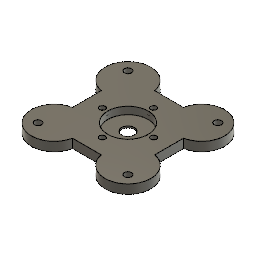
Rotation Motor Top Mount (Autodesk Fusion 360 design; units mm, degrees)
Autodesk Fusion 360 part; units mm, degrees
sketch "Sketch1" plane through (0, 0, 0) normal (0, 1, 0) x (1, 0, 0)
  line L0 (22.5, -7.87) -> (22.5, 7.87)
  circle A0 centre (24.5659, 24.5659) radius 1.95
  arc A1 (22.5, 7.87) -> (7.87, 22.5) centre (20.1464, 20.1464) ccw
  circle A2 centre (24.5659, -24.5659) radius 1.95
  arc A3 (7.87, -22.5) -> (22.5, -7.87) centre (20.1464, -20.1464) ccw
  arc A4 (-7.87, 22.5) -> (-22.5, 7.87) centre (-20.1464, 20.1464) ccw
  line L1 (7.87, 22.5) -> (-7.87, 22.5)
  arc A5 (-22.5, -7.87) -> (-7.87, -22.5) centre (-20.1464, -20.1464) ccw
  line L2 (-7.87, -22.5) -> (7.87, -22.5)
  line L3 (-22.5, 7.87) -> (-22.5, -7.87)
  circle A6 centre (-24.5659, -24.5659) radius 1.95
  circle A7 centre (-24.5659, 24.5659) radius 1.95
  circle A8 centre (0, 0) radius 14
  circle A9 centre (0, -14) radius 1.55
  circle A10 centre (0, -14) radius 2.75
  circle A11 centre (14, 0) radius 2.75
  circle A12 centre (14, 0) radius 1.55
  circle A13 centre (0, 14) radius 2.75
  circle A14 centre (0, 14) radius 1.55
  circle A15 centre (-14, 0) radius 2.75
  circle A16 centre (-14, 0) radius 1.55
  circle A17 centre (0, 0) radius 3.5
  circle A18 centre (0, 0) radius 11.05
  dimension "d1" = 28
  dimension "d2" = 3.1
  dimension "d3" = 5.5
  dimension "d5" = 360
  dimension "d13" = 7
  dimension "d14" = 22.1
  constraint coincident A8.centre A17.centre
  constraint coincident A8 A9.centre
  constraint concentric A9 A10
  constraint concentric A8 A18
  measures "d1" diameter of A8
  measures "d2" diameter of A9
  measures "d3" diameter of A10
  measures "d13" diameter of A17
  measures "d14" diameter of A18
extrude "Extrude1" add sketch "Sketch1" along normal blind 5 contours L0 A1 A3 A4 L1 A5 L2 L3 | A8 A11 A12 | A8 A11 A12 | A8 A10 A11 A13 A15 | A8 A13 A14 | A8 A13 A14 | A8 A9 A10 | A8 A9 A10 | A8 A15 A16 | A8 A15 A16 | A18
extrude "Extrude2" cut sketch "Sketch1" along normal blind 3 contours A8 A11 A12 | A8 A11 A12 | A8 A13 A14 | A8 A13 A14 | A8 A9 A10 | A8 A9 A10 | A8 A15 A16 | A8 A15 A16
extrude "Extrude3" cut sketch "Sketch1" against normal blind 3 from surface at 5 contours A18
extrude "Extrude4" cut 1 faces at (8.4922, 2, 0.549) along direction (0, -1, 0) blind 1
